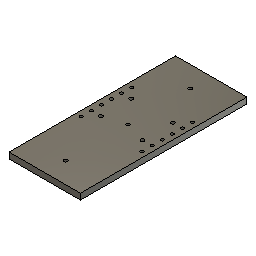
plywood_plate v12 (Autodesk Fusion 360 design; units mm, degrees)
Autodesk Fusion 360 part; units mm, degrees
sketch "Sketch1" plane through (0, 0, 0) normal (0, 1, 0) x (1, 0, 0)
  line L0 (60, 140) -> (-60, 140)
  line L1 (-60, 140) -> (-60, -140)
  line L2 (-60, -140) -> (60, -140)
  line L3 (60, -140) -> (60, 140)
  line L4 (60, 140) -> (-60, -140) construction
  line L5 (-60, 140) -> (60, -140) construction
  line L6 (0, 160) -> (0, -180) construction
  line L7 (-113.0657, 15) -> (80.2615, 15) construction
  line L8 (80.2615, 15) -> (130.9595, 14.8382) construction
  line L9 (130.9595, 14.8382) -> (130.9763, 20.0945) construction
  line L10 (130.9763, 20.0945) -> (80.2783, 20.2563) construction
  line L11 (80.2783, 20.2563) -> (80.2615, 15) construction
  circle A0 centre (0, -105) radius 3
  circle A1 centre (0, 0) radius 3
  line L12 (-100.8455, 0) -> (89.1545, 0) construction
  circle A2 centre (0, 105) radius 3
  circle A3 centre (51, 23.5) radius 2.5
  circle A4 centre (51, 40.5) radius 2.5
  circle A5 centre (51, 57.5) radius 2.5
  line L13 (51, 19.633) -> (51, 57.5)
  line L14 (60, 40.5) -> (35, 40.5)
  circle A6 centre (35, 40.5) radius 3
  circle A7 centre (51, 6.5) radius 2.5
  circle A8 centre (51, -10.5) radius 2.5
  circle A9 centre (51, -27.5) radius 2.5
  circle A10 centre (35, -10.5) radius 3
  circle A11 centre (-35, -10.5) radius 3
  circle A12 centre (-51, -10.5) radius 2.5
  circle A13 centre (-51, 6.5) radius 2.5
  circle A14 centre (-51, 23.5) radius 2.5
  circle A15 centre (-51, 40.5) radius 2.5
  circle A16 centre (-51, 57.5) radius 2.5
  circle A17 centre (-35, 40.5) radius 3
  circle A18 centre (-51, -27.5) radius 2.5
  dimension "d1" = 120
  dimension "d2" = 280
  dimension "d3" = 5
  dimension "d4" = 155
  dimension "d5" = 6
  dimension "d6" = 35
  dimension "d7" = 6
  dimension "d11" = 5
  dimension "d12" = 9
  dimension "d14" = 5
  dimension "d15" = 17
  dimension "d16" = 5
  dimension "d17" = 17
  dimension "d18" = 25
  dimension "d19" = 6
  dimension "d20" = 8.5
  dimension "d21" = 15
  constraint horizontal L0
  constraint perpendicular L0 L1
  constraint parallel L0 L2
  constraint parallel L1 L3
  constraint coincident L4 A1.centre
  constraint coincident L5 A1.centre
  constraint coincident A1.centre origin
  constraint perpendicular L2 L6
  constraint coincident L7.end
  constraint coincident L6 A0.centre
  constraint coincident L6 A1.centre
  constraint perpendicular L3 L12
  constraint coincident A1.centre L12
  constraint coincident A1.centre L6
  constraint symmetric A0 L12 A2
  constraint coincident A5.centre L13.end
  constraint coincident A3.centre L13
  constraint coincident A4.centre L13
  constraint coincident L3 L14.start
  constraint perpendicular L3 L14
  constraint coincident L14.end A6.centre
  constraint coincident A4.centre L14
  constraint perpendicular L7 L13
  constraint symmetric L7 A3 A7
  constraint symmetric L7 A4 A8
  constraint symmetric L7 A5 A9
  constraint symmetric L7 A6 A10
  constraint symmetric L6 A3 A14
  constraint symmetric L6 A4 A15
  constraint symmetric L6 A5 A16
  constraint symmetric L6 A6 A17
  constraint symmetric L6 A7 A13
  constraint symmetric L6 A8 A12
  constraint symmetric L6 A10 A11
  constraint symmetric L6 A9 A18
  measures "d1" distance of L1.end L2.end
  measures "d2" distance of L0.end L1.end
  measures "d4" distance of L2 L7
  measures "d5" diameter of A0
  measures "d6" distance of L2 A0.centre
  measures "d7" diameter of A1
  measures "d11" diameter of A3
  measures "d12" distance of L3 A3.centre
  measures "d14" diameter of A4
  measures "d15" distance of A3.centre A4.centre
  measures "d16" diameter of A5
  measures "d17" distance of A4.centre A5.centre
  measures "d18" distance of L14.start L14.end
  measures "d19" diameter of A6
  measures "d20" distance of L7 A3.centre
  measures "d21" distance of L7 L12
extrude "Extrude1" add sketch "Sketch1" along normal blind 10
equation "d18 = 22.00 mm + ( d19 / 2 mm ) * 1 mm"
